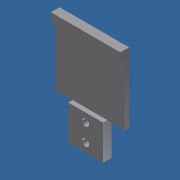
# Autodesk Inventor part: gripper jaw extension
Saved by Autodesk Inventor 2012 (Build 160160000, 160)
## iProperties
Created: 2012-07-09
Part Number: gripper jaw extension
Material: Default
Document SubType Name: Modeling
Designer: Ed
Density: 1 g/cm^3
Author: Ed
Autodesk Inventor part; units mm, degrees
ref_plane "YZ Plane" through (0, 0, 0) normal (1, 0, 0) x (0, 1, 0)
ref_plane "XZ Plane" through (0, 0, 0) normal (0, 1, 0) x (-1, 0, 0)
ref_plane "XY Plane" through (0, 0, 0) normal (0, 0, 1) x (1, 0, 0)
sketch "Sketch1" plane through (0, 0, 0) normal (0, 0, 1) x (1, 0, 0)
  line L0 (-12.7, 0) -> (12.7, 0)
  line L1 (12.7, 0) -> (12.7, 25.4)
  line L2 (12.7, 25.4) -> (-12.7, 25.4)
  line L3 (-12.7, 25.4) -> (-12.7, 0)
  line L4 (-25.4, 25.4) -> (25.4, 25.4)
  line L5 (25.4, 25.4) -> (25.4, 76.2)
  line L6 (25.4, 76.2) -> (-25.4, 76.2)
  line L7 (-25.4, 76.2) -> (-25.4, 25.4)
  point P0 (0, 0)
  point P1 (0, 25.4)
  point P2 (0, 0)
  dimension "d0" = 25.4
  dimension "d1" = 50.8
  dimension "d2" = 25.4
  dimension "d3" = 50.8
  constraints: 16 end point, 4 parallel, 3 midpoint, 2 horizontal, 2 perpendicular, 1 coincident
  measures "d0" distance of L0.start L0.end
  measures "d1" distance of L5.end L6.end
  measures "d2" distance of L0.end L1.end
  measures "d3" distance of L4.end L5.end
extrude "Extrusion1" add sketch "Sketch1" along normal blind 3.175
sketch "Sketch2" plane through (0, 0, 3.175) normal (0, 0, 1) x (1, 0, 0)
  line L0 (-12.7, 0) -> (12.7, 0)
  line L1 (12.7, 0) -> (12.7, 25.4)
  line L2 (12.7, 25.4) -> (-12.7, 25.4)
  line L3 (-12.7, 25.4) -> (-12.7, 0)
  line L4 (25.4, 76.2) -> (25.4, 25.4) projected
  line L5 (-25.4, 76.2) -> (25.4, 76.2) projected
  line L6 (-25.4, 76.2) -> (25.4, 76.2)
  line L7 (25.4, 76.2) -> (25.4, 69.85)
  line L8 (25.4, 69.85) -> (-25.4, 69.85)
  line L9 (-25.4, 69.85) -> (-25.4, 76.2)
  line L10 (-12.7, 0) -> (-12.7, 25.4) projected
  line L11 (12.7, 25.4) -> (12.7, 0) projected
  line L12 (25.4, 25.4) -> (12.7, 25.4) projected
  line L13 (-12.7, 25.4) -> (-25.4, 25.4) projected
  line L14 (-12.7, 25.4) -> (-13.5255, 25.4)
  arc A0 (-12.7, 24.5745) -> (-13.5255, 25.4) centre (-13.5255, 24.5745) ccw
  line L15 (12.7, 25.4) -> (13.5255, 25.4)
  arc A1 (13.5255, 25.4) -> (12.7, 24.5745) centre (13.5255, 24.5745) ccw
  point P0 (0, 0)
  dimension "d17" = 6.35
  dimension "d19" = 0.8255
  constraints: 20 end point, 5 point on line, 4 parallel, 4 point on circle, 3 tangent, 2 centre point, 2 horizontal, 2 perpendicular, 1 collinear, 1 equal radius
  measures "d17" distance between parallel lines of L5 L8
  measures "d19" radius of A1
extrude "Extrusion2" add sketch "Sketch2" along normal blind 3.175 contours L3 L2 L1 L0 | L8 L9 L5 L4
fillet "Fillet1" radius 1.5875 2 edges at (12.7, 25.4, 1.5875) (-12.7, 25.4, 1.5875)
sketch "Sketch3" plane through (0, 0, 0) normal (0, 0, -1) x (-1, 0, 0)
  line L0 (12.7, 0) -> (-12.7, 0) projected
  point P0 (0, 0)
  point P1 (0, 6.35)
  point P2 (0, 19.05)
  point P3 (0, 0)
  dimension "d8" = 12.7
  dimension "d9" = 6.35
  constraints: 2 vertical alignment, 1 midpoint
  measures "d8" distance of point (0, 19.05) point (0, 6.35)
  measures "d9" distance of point (0, 0) point (0, 6.35)
hole "Hole1" at (0, 6.35, 0) at (0, 19.05, 0) direction (0, 0, 1) diameter 5.1054 end through all clearance for "Flat Head Machine Screw (82)" size "#10" standard "Ansi Unified Screw Threads"
body "Solid1"
